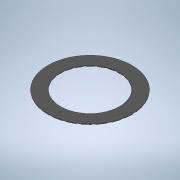
# Autodesk Inventor part: Tarcza_Okładzina_Cierna
Saved by Autodesk Inventor 2022 (Build 260153000, 153)
## iProperties
Created: 2021-06-19
Part Number: Tarcza_Okładzina_Cierna
Material: Kevlar49
Document SubType Name: Modeling
Designer: Matik
Density: 0.052 g/cm^3
Appearance: Ogólny
Author: Matik
Autodesk Inventor part; units mm, degrees
ref_plane "YZ Plane" through (0, 0, 0) normal (1, 0, 0) x (0, 1, 0)
ref_plane "XZ Plane" through (0, 0, 0) normal (0, 1, 0) x (-1, 0, 0)
ref_plane "XY Plane" through (0, 0, 0) normal (0, 0, 1) x (1, 0, 0)
sketch "Szkic1" plane through (0, 0, 0) normal (0, 1, 0) x (-1, 0, 0)
  circle A0 centre (0, 0) radius 100
  circle A1 centre (0, 0) radius 70
  line L0 (70, 0) -> (70, 5.198254)
  line L1 (70, 0) -> (70, -6.043615)
  line L2 (72.279206, 7.178669) -> (98.104364, 3.537745)
  line L3 (71.386072, -7.947058) -> (96.155566, -15.936103)
  line L4 (99.820589, 1.422211) -> (98.764925, -14.16778)
  arc A2 (72.279206, 7.178669) -> (70, 5.198254) centre (72, 5.198254) ccw
  arc A3 (70, -6.043615) -> (71.386072, -7.947058) centre (72, -6.043615) ccw
  arc A4 (96.155566, -15.936103) -> (98.764925, -14.16778) centre (96.769494, -14.032661) ccw
  arc A5 (99.820589, 1.422211) -> (98.104364, 3.537745) centre (97.825158, 1.55733) ccw
  line L5 (96.051189, 27.20922) -> (99.066483, 11.877219)
  arc A6 (96.051189, 27.20922) -> (93.845903, 28.808478) centre (94.08878, 26.82328) ccw
  line L6 (67.958375, 25.641297) -> (93.845903, 28.808478)
  arc A7 (67.958375, 25.641297) -> (66.269401, 23.138461) centre (68.201252, 23.656099) ccw
  line L7 (67.614808, 18.117333) -> (69.179011, 12.279649)
  line L8 (67.614808, 18.117333) -> (66.269401, 23.138461)
  line L9 (71.0105, 10.799807) -> (97.003712, 9.493798)
  arc A8 (69.179011, 12.279649) -> (71.0105, 10.799807) centre (71.110862, 12.797287) ccw
  arc A9 (97.003712, 9.493798) -> (99.066483, 11.877219) centre (97.104074, 11.491278) ccw
  line L10 (85.73606, 51.141966) -> (92.616824, 37.112805)
  arc A10 (85.73606, 51.141966) -> (83.191999, 52.11596) centre (83.940407, 50.261267) ccw
  line L11 (59.006294, 42.356513) -> (83.191999, 52.11596)
  arc A11 (59.006294, 42.356513) -> (58.022651, 39.50182) centre (59.754702, 40.50182) ccw
  line L12 (60.621778, 35) -> (63.643586, 29.766076)
  line L13 (60.621778, 35) -> (58.022651, 39.50182)
  line L14 (65.795681, 28.810682) -> (91.241215, 34.276713)
  arc A12 (63.643586, 29.766076) -> (65.795681, 28.810682) centre (65.375637, 30.766076) ccw
  arc A13 (91.241215, 34.276713) -> (92.616824, 37.112805) centre (90.821171, 36.232106) ccw
  line L15 (69.57816, 71.589471) -> (79.855481, 59.819215)
  arc A14 (69.57816, 71.589471) -> (66.868698, 71.871825) centre (68.071634, 70.274032) ccw
  line L16 (46.033031, 56.185202) -> (66.868698, 71.871825)
  arc A15 (46.033031, 56.185202) -> (45.821754, 53.173195) centre (47.235967, 54.587409) ccw
  line L17 (49.497475, 49.497475) -> (53.770956, 45.223993)
  line L18 (49.497475, 49.497475) -> (45.821754, 53.173195)
  line L19 (56.096994, 44.858157) -> (79.26078, 56.723726)
  arc A16 (53.770956, 45.223993) -> (56.096994, 44.858157) centre (55.18517, 46.638207) ccw
  arc A17 (79.26078, 56.723726) -> (79.855481, 59.819215) centre (78.348955, 58.503776) ccw
  line L20 (48.678623, 87.158271) -> (61.65212, 78.449044)
  arc A18 (48.678623, 87.158271) -> (45.988405, 86.729745) centre (47.563892, 85.497737) ccw
  line L21 (29.922693, 66.184963) -> (45.988405, 86.729745)
  arc A19 (29.922693, 66.184963) -> (30.49818, 63.220905) centre (31.49818, 64.952956) ccw
  line L22 (35, 60.621778) -> (40.233924, 57.599971)
  line L23 (35, 60.621778) -> (30.49818, 63.220905)
  line L24 (42.57539, 57.848623) -> (61.878853, 75.305111)
  arc A20 (40.233924, 57.599971) -> (42.57539, 57.848623) centre (41.233924, 59.332021) ccw
  arc A21 (61.878853, 75.305111) -> (61.65212, 78.449044) centre (60.537388, 76.78851) ccw
  line L25 (24.461719, 96.78738) -> (39.247268, 91.7327)
  arc A22 (24.461719, 96.78738) -> (21.974078, 95.677175) centre (23.814749, 94.894914) ccw
  line L26 (11.773173, 71.674328) -> (21.974078, 95.677175)
  arc A23 (11.773173, 71.674328) -> (13.096205, 68.960215) centre (13.613843, 70.892067) ccw
  line L27 (18.117333, 67.614808) -> (23.955017, 66.050605)
  line L28 (18.117333, 67.614808) -> (13.096205, 68.960215)
  line L29 (26.152343, 66.896801) -> (40.279986, 88.754578)
  arc A24 (23.955017, 66.050605) -> (26.152343, 66.896801) centre (24.472655, 67.982457) ccw
  arc A25 (40.279986, 88.754578) -> (39.247268, 91.7327) centre (38.600298, 89.840234) ccw
  line L30 (-1.422211, 99.820589) -> (14.16778, 98.764925)
  arc A26 (-1.422211, 99.820589) -> (-3.537745, 98.104364) centre (-1.55733, 97.825158) ccw
  line L31 (-7.178669, 72.279206) -> (-3.537745, 98.104364)
  arc A27 (-7.178669, 72.279206) -> (-5.198254, 70) centre (-5.198254, 72) ccw
  line L32 (0, 70) -> (6.043615, 70)
  line L33 (0, 70) -> (-5.198254, 70)
  line L34 (7.947058, 71.386072) -> (15.936103, 96.155566)
  arc A28 (6.043615, 70) -> (7.947058, 71.386072) centre (6.043615, 72) ccw
  arc A29 (15.936103, 96.155566) -> (14.16778, 98.764925) centre (14.032661, 96.769494) ccw
  line L35 (-27.20922, 96.051189) -> (-11.877219, 99.066483)
  arc A30 (-27.20922, 96.051189) -> (-28.808478, 93.845903) centre (-26.82328, 94.08878) ccw
  line L36 (-25.641297, 67.958375) -> (-28.808478, 93.845903)
  arc A31 (-25.641297, 67.958375) -> (-23.138461, 66.269401) centre (-23.656099, 68.201252) ccw
  line L37 (-18.117333, 67.614808) -> (-12.279649, 69.179011)
  line L38 (-18.117333, 67.614808) -> (-23.138461, 66.269401)
  line L39 (-10.799807, 71.0105) -> (-9.493798, 97.003712)
  arc A32 (-12.279649, 69.179011) -> (-10.799807, 71.0105) centre (-12.797287, 71.110862) ccw
  arc A33 (-9.493798, 97.003712) -> (-11.877219, 99.066483) centre (-11.491278, 97.104074) ccw
  line L40 (-51.141966, 85.73606) -> (-37.112805, 92.616824)
  arc A34 (-51.141966, 85.73606) -> (-52.11596, 83.191999) centre (-50.261267, 83.940407) ccw
  line L41 (-42.356513, 59.006294) -> (-52.11596, 83.191999)
  arc A35 (-42.356513, 59.006294) -> (-39.50182, 58.022651) centre (-40.50182, 59.754702) ccw
  line L42 (-35, 60.621778) -> (-29.766076, 63.643586)
  line L43 (-35, 60.621778) -> (-39.50182, 58.022651)
  line L44 (-28.810682, 65.795681) -> (-34.276713, 91.241215)
  arc A36 (-29.766076, 63.643586) -> (-28.810682, 65.795681) centre (-30.766076, 65.375637) ccw
  arc A37 (-34.276713, 91.241215) -> (-37.112805, 92.616824) centre (-36.232106, 90.821171) ccw
  line L45 (-71.589471, 69.57816) -> (-59.819215, 79.855481)
  arc A38 (-71.589471, 69.57816) -> (-71.871825, 66.868698) centre (-70.274032, 68.071634) ccw
  line L46 (-56.185202, 46.033031) -> (-71.871825, 66.868698)
  arc A39 (-56.185202, 46.033031) -> (-53.173195, 45.821754) centre (-54.587409, 47.235967) ccw
  line L47 (-49.497475, 49.497475) -> (-45.223993, 53.770956)
  line L48 (-49.497475, 49.497475) -> (-53.173195, 45.821754)
  line L49 (-44.858157, 56.096994) -> (-56.723726, 79.26078)
  arc A40 (-45.223993, 53.770956) -> (-44.858157, 56.096994) centre (-46.638207, 55.18517) ccw
  arc A41 (-56.723726, 79.26078) -> (-59.819215, 79.855481) centre (-58.503776, 78.348955) ccw
  line L50 (-87.158271, 48.678623) -> (-78.449044, 61.65212)
  arc A42 (-87.158271, 48.678623) -> (-86.729745, 45.988405) centre (-85.497737, 47.563892) ccw
  line L51 (-66.184963, 29.922693) -> (-86.729745, 45.988405)
  arc A43 (-66.184963, 29.922693) -> (-63.220905, 30.49818) centre (-64.952956, 31.49818) ccw
  line L52 (-60.621778, 35) -> (-57.599971, 40.233924)
  line L53 (-60.621778, 35) -> (-63.220905, 30.49818)
  line L54 (-57.848623, 42.57539) -> (-75.305111, 61.878853)
  arc A44 (-57.599971, 40.233924) -> (-57.848623, 42.57539) centre (-59.332021, 41.233924) ccw
  arc A45 (-75.305111, 61.878853) -> (-78.449044, 61.65212) centre (-76.78851, 60.537388) ccw
  line L55 (-96.78738, 24.461719) -> (-91.7327, 39.247268)
  arc A46 (-96.78738, 24.461719) -> (-95.677175, 21.974078) centre (-94.894914, 23.814749) ccw
  line L56 (-71.674328, 11.773173) -> (-95.677175, 21.974078)
  arc A47 (-71.674328, 11.773173) -> (-68.960215, 13.096205) centre (-70.892067, 13.613843) ccw
  line L57 (-67.614808, 18.117333) -> (-66.050605, 23.955017)
  line L58 (-67.614808, 18.117333) -> (-68.960215, 13.096205)
  line L59 (-66.896801, 26.152343) -> (-88.754578, 40.279986)
  arc A48 (-66.050605, 23.955017) -> (-66.896801, 26.152343) centre (-67.982457, 24.472655) ccw
  arc A49 (-88.754578, 40.279986) -> (-91.7327, 39.247268) centre (-89.840234, 38.600298) ccw
  line L60 (-99.820589, -1.422211) -> (-98.764925, 14.16778)
  arc A50 (-99.820589, -1.422211) -> (-98.104364, -3.537745) centre (-97.825158, -1.55733) ccw
  line L61 (-72.279206, -7.178669) -> (-98.104364, -3.537745)
  arc A51 (-72.279206, -7.178669) -> (-70, -5.198254) centre (-72, -5.198254) ccw
  line L62 (-70, 0) -> (-70, 6.043615)
  line L63 (-70, 0) -> (-70, -5.198254)
  line L64 (-71.386072, 7.947058) -> (-96.155566, 15.936103)
  arc A52 (-70, 6.043615) -> (-71.386072, 7.947058) centre (-72, 6.043615) ccw
  arc A53 (-96.155566, 15.936103) -> (-98.764925, 14.16778) centre (-96.769494, 14.032661) ccw
  line L65 (-96.051189, -27.20922) -> (-99.066483, -11.877219)
  arc A54 (-96.051189, -27.20922) -> (-93.845903, -28.808478) centre (-94.08878, -26.82328) ccw
  line L66 (-67.958375, -25.641297) -> (-93.845903, -28.808478)
  arc A55 (-67.958375, -25.641297) -> (-66.269401, -23.138461) centre (-68.201252, -23.656099) ccw
  line L67 (-67.614808, -18.117333) -> (-69.179011, -12.279649)
  line L68 (-67.614808, -18.117333) -> (-66.269401, -23.138461)
  line L69 (-71.0105, -10.799807) -> (-97.003712, -9.493798)
  arc A56 (-69.179011, -12.279649) -> (-71.0105, -10.799807) centre (-71.110862, -12.797287) ccw
  arc A57 (-97.003712, -9.493798) -> (-99.066483, -11.877219) centre (-97.104074, -11.491278) ccw
  line L70 (-85.73606, -51.141966) -> (-92.616824, -37.112805)
  arc A58 (-85.73606, -51.141966) -> (-83.191999, -52.11596) centre (-83.940407, -50.261267) ccw
  line L71 (-59.006294, -42.356513) -> (-83.191999, -52.11596)
  arc A59 (-59.006294, -42.356513) -> (-58.022651, -39.50182) centre (-59.754702, -40.50182) ccw
  line L72 (-60.621778, -35) -> (-63.643586, -29.766076)
  line L73 (-60.621778, -35) -> (-58.022651, -39.50182)
  line L74 (-65.795681, -28.810682) -> (-91.241215, -34.276713)
  arc A60 (-63.643586, -29.766076) -> (-65.795681, -28.810682) centre (-65.375637, -30.766076) ccw
  arc A61 (-91.241215, -34.276713) -> (-92.616824, -37.112805) centre (-90.821171, -36.232106) ccw
  line L75 (-69.57816, -71.589471) -> (-79.855481, -59.819215)
  arc A62 (-69.57816, -71.589471) -> (-66.868698, -71.871825) centre (-68.071634, -70.274032) ccw
  line L76 (-46.033031, -56.185202) -> (-66.868698, -71.871825)
  arc A63 (-46.033031, -56.185202) -> (-45.821754, -53.173195) centre (-47.235967, -54.587409) ccw
  line L77 (-49.497475, -49.497475) -> (-53.770956, -45.223993)
  line L78 (-49.497475, -49.497475) -> (-45.821754, -53.173195)
  line L79 (-56.096994, -44.858157) -> (-79.26078, -56.723726)
  arc A64 (-53.770956, -45.223993) -> (-56.096994, -44.858157) centre (-55.18517, -46.638207) ccw
  arc A65 (-79.26078, -56.723726) -> (-79.855481, -59.819215) centre (-78.348955, -58.503776) ccw
  line L80 (-48.678623, -87.158271) -> (-61.65212, -78.449044)
  arc A66 (-48.678623, -87.158271) -> (-45.988405, -86.729745) centre (-47.563892, -85.497737) ccw
  line L81 (-29.922693, -66.184963) -> (-45.988405, -86.729745)
  arc A67 (-29.922693, -66.184963) -> (-30.49818, -63.220905) centre (-31.49818, -64.952956) ccw
  line L82 (-35, -60.621778) -> (-40.233924, -57.599971)
  line L83 (-35, -60.621778) -> (-30.49818, -63.220905)
  line L84 (-42.57539, -57.848623) -> (-61.878853, -75.305111)
  arc A68 (-40.233924, -57.599971) -> (-42.57539, -57.848623) centre (-41.233924, -59.332021) ccw
  arc A69 (-61.878853, -75.305111) -> (-61.65212, -78.449044) centre (-60.537388, -76.78851) ccw
  line L85 (-24.461719, -96.78738) -> (-39.247268, -91.7327)
  arc A70 (-24.461719, -96.78738) -> (-21.974078, -95.677175) centre (-23.814749, -94.894914) ccw
  line L86 (-11.773173, -71.674328) -> (-21.974078, -95.677175)
  arc A71 (-11.773173, -71.674328) -> (-13.096205, -68.960215) centre (-13.613843, -70.892067) ccw
  line L87 (-18.117333, -67.614808) -> (-23.955017, -66.050605)
  line L88 (-18.117333, -67.614808) -> (-13.096205, -68.960215)
  line L89 (-26.152343, -66.896801) -> (-40.279986, -88.754578)
  arc A72 (-23.955017, -66.050605) -> (-26.152343, -66.896801) centre (-24.472655, -67.982457) ccw
  arc A73 (-40.279986, -88.754578) -> (-39.247268, -91.7327) centre (-38.600298, -89.840234) ccw
  line L90 (1.422211, -99.820589) -> (-14.16778, -98.764925)
  arc A74 (1.422211, -99.820589) -> (3.537745, -98.104364) centre (1.55733, -97.825158) ccw
  line L91 (7.178669, -72.279206) -> (3.537745, -98.104364)
  arc A75 (7.178669, -72.279206) -> (5.198254, -70) centre (5.198254, -72) ccw
  line L92 (0, -70) -> (-6.043615, -70)
  line L93 (0, -70) -> (5.198254, -70)
  line L94 (-7.947058, -71.386072) -> (-15.936103, -96.155566)
  arc A76 (-6.043615, -70) -> (-7.947058, -71.386072) centre (-6.043615, -72) ccw
  arc A77 (-15.936103, -96.155566) -> (-14.16778, -98.764925) centre (-14.032661, -96.769494) ccw
  line L95 (27.20922, -96.051189) -> (11.877219, -99.066483)
  arc A78 (27.20922, -96.051189) -> (28.808478, -93.845903) centre (26.82328, -94.08878) ccw
  line L96 (25.641297, -67.958375) -> (28.808478, -93.845903)
  arc A79 (25.641297, -67.958375) -> (23.138461, -66.269401) centre (23.656099, -68.201252) ccw
  line L97 (18.117333, -67.614808) -> (12.279649, -69.179011)
  line L98 (18.117333, -67.614808) -> (23.138461, -66.269401)
  line L99 (10.799807, -71.0105) -> (9.493798, -97.003712)
  arc A80 (12.279649, -69.179011) -> (10.799807, -71.0105) centre (12.797287, -71.110862) ccw
  arc A81 (9.493798, -97.003712) -> (11.877219, -99.066483) centre (11.491278, -97.104074) ccw
  line L100 (51.141966, -85.73606) -> (37.112805, -92.616824)
  arc A82 (51.141966, -85.73606) -> (52.11596, -83.191999) centre (50.261267, -83.940407) ccw
  line L101 (42.356513, -59.006294) -> (52.11596, -83.191999)
  arc A83 (42.356513, -59.006294) -> (39.50182, -58.022651) centre (40.50182, -59.754702) ccw
  line L102 (35, -60.621778) -> (29.766076, -63.643586)
  line L103 (35, -60.621778) -> (39.50182, -58.022651)
  line L104 (28.810682, -65.795681) -> (34.276713, -91.241215)
  arc A84 (29.766076, -63.643586) -> (28.810682, -65.795681) centre (30.766076, -65.375637) ccw
  arc A85 (34.276713, -91.241215) -> (37.112805, -92.616824) centre (36.232106, -90.821171) ccw
  line L105 (71.589471, -69.57816) -> (59.819215, -79.855481)
  arc A86 (71.589471, -69.57816) -> (71.871825, -66.868698) centre (70.274032, -68.071634) ccw
  line L106 (56.185202, -46.033031) -> (71.871825, -66.868698)
  arc A87 (56.185202, -46.033031) -> (53.173195, -45.821754) centre (54.587409, -47.235967) ccw
  line L107 (49.497475, -49.497475) -> (45.223993, -53.770956)
  line L108 (49.497475, -49.497475) -> (53.173195, -45.821754)
  line L109 (44.858157, -56.096994) -> (56.723726, -79.26078)
  arc A88 (45.223993, -53.770956) -> (44.858157, -56.096994) centre (46.638207, -55.18517) ccw
  arc A89 (56.723726, -79.26078) -> (59.819215, -79.855481) centre (58.503776, -78.348955) ccw
  line L110 (87.158271, -48.678623) -> (78.449044, -61.65212)
  arc A90 (87.158271, -48.678623) -> (86.729745, -45.988405) centre (85.497737, -47.563892) ccw
  line L111 (66.184963, -29.922693) -> (86.729745, -45.988405)
  arc A91 (66.184963, -29.922693) -> (63.220905, -30.49818) centre (64.952956, -31.49818) ccw
  line L112 (60.621778, -35) -> (57.599971, -40.233924)
  line L113 (60.621778, -35) -> (63.220905, -30.49818)
  line L114 (57.848623, -42.57539) -> (75.305111, -61.878853)
  arc A92 (57.599971, -40.233924) -> (57.848623, -42.57539) centre (59.332021, -41.233924) ccw
  arc A93 (75.305111, -61.878853) -> (78.449044, -61.65212) centre (76.78851, -60.537388) ccw
  line L115 (96.78738, -24.461719) -> (91.7327, -39.247268)
  arc A94 (96.78738, -24.461719) -> (95.677175, -21.974078) centre (94.894914, -23.814749) ccw
  line L116 (71.674328, -11.773173) -> (95.677175, -21.974078)
  arc A95 (71.674328, -11.773173) -> (68.960215, -13.096205) centre (70.892067, -13.613843) ccw
  line L117 (67.614808, -18.117333) -> (66.050605, -23.955017)
  line L118 (67.614808, -18.117333) -> (68.960215, -13.096205)
  line L119 (66.896801, -26.152343) -> (88.754578, -40.279986)
  arc A96 (66.050605, -23.955017) -> (66.896801, -26.152343) centre (67.982457, -24.472655) ccw
  arc A97 (88.754578, -40.279986) -> (91.7327, -39.247268) centre (89.840234, -38.600298) ccw
  point P0 (70, 7.5)
  point P1 (70, -7.5)
  point P2 (99.946257, 3.278069)
  point P3 (98.591972, -16.721931)
  point P4 (98.591972, -16.721931)
  point P5 (99.560487, 9.365335)
  point P6 (95.692244, 29.034366)
  point P7 (65.673665, 25.361777)
  point P8 (69.555951, 10.872889)
  point P9 (99.560487, 9.365335)
  point P10 (93.744118, 34.814369)
  point P11 (84.916963, 52.812019)
  point P12 (56.871778, 41.495191)
  point P13 (64.371778, 28.504809)
  point P14 (93.744118, 34.814369)
  point P15 (81.539243, 57.890861)
  point P16 (68.354731, 72.990621)
  point P17 (44.194174, 54.800776)
  point P18 (54.800776, 44.194174)
  point P19 (81.539243, 57.890861)
  point P20 (63.777603, 77.022187)
  point P21 (47.134238, 88.195032)
  point P22 (28.504809, 64.371778)
  point P23 (41.495191, 56.871778)
  point P24 (63.777603, 77.022187)
  point P25 (41.669625, 90.904578)
  point P26 (22.701623, 97.389097)
  point P27 (10.872889, 69.555951)
  point P28 (25.361777, 65.673665)
  point P29 (41.669625, 90.904578)
  point P30 (16.721931, 98.591972)
  point P31 (-3.278069, 99.946257)
  point P32 (-7.5, 70)
  point P33 (7.5, 70)
  point P34 (16.721931, 98.591972)
  point P35 (-9.365335, 99.560487)
  point P36 (-29.034366, 95.692244)
  point P37 (-25.361777, 65.673665)
  point P38 (-10.872889, 69.555951)
  point P39 (-9.365335, 99.560487)
  point P40 (-34.814369, 93.744118)
  point P41 (-52.812019, 84.916963)
  point P42 (-41.495191, 56.871778)
  point P43 (-28.504809, 64.371778)
  point P44 (-34.814369, 93.744118)
  point P45 (-57.890861, 81.539243)
  point P46 (-72.990621, 68.354731)
  point P47 (-54.800776, 44.194174)
  point P48 (-44.194174, 54.800776)
  point P49 (-57.890861, 81.539243)
  point P50 (-77.022187, 63.777603)
  point P51 (-88.195032, 47.134238)
  point P52 (-64.371778, 28.504809)
  point P53 (-56.871778, 41.495191)
  point P54 (-77.022187, 63.777603)
  point P55 (-90.904578, 41.669625)
  point P56 (-97.389097, 22.701623)
  point P57 (-69.555951, 10.872889)
  point P58 (-65.673665, 25.361777)
  point P59 (-90.904578, 41.669625)
  point P60 (-98.591972, 16.721931)
  point P61 (-99.946257, -3.278069)
  point P62 (-70, -7.5)
  point P63 (-70, 7.5)
  point P64 (-98.591972, 16.721931)
  point P65 (-99.560487, -9.365335)
  point P66 (-95.692244, -29.034366)
  point P67 (-65.673665, -25.361777)
  point P68 (-69.555951, -10.872889)
  point P69 (-99.560487, -9.365335)
  point P70 (-93.744118, -34.814369)
  point P71 (-84.916963, -52.812019)
  point P72 (-56.871778, -41.495191)
  point P73 (-64.371778, -28.504809)
  point P74 (-93.744118, -34.814369)
  point P75 (-81.539243, -57.890861)
  point P76 (-68.354731, -72.990621)
  point P77 (-44.194174, -54.800776)
  point P78 (-54.800776, -44.194174)
  point P79 (-81.539243, -57.890861)
  point P80 (-63.777603, -77.022187)
  point P81 (-47.134238, -88.195032)
  point P82 (-28.504809, -64.371778)
  point P83 (-41.495191, -56.871778)
  point P84 (-63.777603, -77.022187)
  point P85 (-41.669625, -90.904578)
  point P86 (-22.701623, -97.389097)
  point P87 (-10.872889, -69.555951)
  point P88 (-25.361777, -65.673665)
  point P89 (-41.669625, -90.904578)
  point P90 (-16.721931, -98.591972)
  point P91 (3.278069, -99.946257)
  point P92 (7.5, -70)
  point P93 (-7.5, -70)
  point P94 (-16.721931, -98.591972)
  point P95 (9.365335, -99.560487)
  point P96 (29.034366, -95.692244)
  point P97 (25.361777, -65.673665)
  point P98 (10.872889, -69.555951)
  point P99 (9.365335, -99.560487)
  point P100 (34.814369, -93.744118)
  point P101 (52.812019, -84.916963)
  point P102 (41.495191, -56.871778)
  point P103 (28.504809, -64.371778)
  point P104 (34.814369, -93.744118)
  point P105 (57.890861, -81.539243)
  point P106 (72.990621, -68.354731)
  point P107 (54.800776, -44.194174)
  point P108 (44.194174, -54.800776)
  point P109 (57.890861, -81.539243)
  point P110 (77.022187, -63.777603)
  point P111 (88.195032, -47.134238)
  point P112 (64.371778, -28.504809)
  point P113 (56.871778, -41.495191)
  point P114 (77.022187, -63.777603)
  point P115 (90.904578, -41.669625)
  point P116 (97.389097, -22.701623)
  point P117 (69.555951, -10.872889)
  point P118 (65.673665, -25.361777)
  point P119 (90.904578, -41.669625)
  dimension "d1" = 140
  dimension "d0" = 200
  dimension "d3" = 7.5
  dimension "d4" = 7.5
  dimension "d7" = 20
  dimension "d8" = 2
  dimension "d11" = 360
  constraints: 240 end point, 216 point on line, 195 point on circle, 97 centre point, 8 tangent, 3 equal radius, 2 coincident, 2 vertical, 1 horizontal alignment, 651 other
  measures "d0" diameter of A0
  measures "d3" distance of L0.start point (70, 7.5)
  measures "d4" distance of L0.start point (70, -7.5)
  measures "d7" vertical distance of point (98.592, -16.722) A0.start
  measures "d8" radius of A2
sketch "Szkic1 outline for Wyciągnięcie proste1" plane through (0, 0, 0) normal (0, 1, 0) x (-1, 0, 0)
  arc A0 (69.179011, 12.279649) -> (71.0105, 10.799807) centre (71.110862, 12.797287) ccw
  line L0 (71.0105, 10.799807) -> (97.003712, 9.493798)
  arc A1 (97.003712, 9.493798) -> (99.066483, 11.877219) centre (97.104074, 11.491278) ccw
  line L1 (99.066483, 11.877219) -> (96.051189, 27.20922)
  arc A2 (96.051189, 27.20922) -> (93.845903, 28.808478) centre (94.08878, 26.82328) ccw
  line L2 (93.845903, 28.808478) -> (67.958375, 25.641297)
  arc A3 (67.958375, 25.641297) -> (66.269401, 23.138461) centre (68.201252, 23.656099) ccw
  line L3 (66.269401, 23.138461) -> (69.179011, 12.279649)
  arc A4 (63.643586, 29.766076) -> (65.795681, 28.810682) centre (65.375637, 30.766076) ccw
  line L4 (65.795681, 28.810682) -> (91.241215, 34.276713)
  arc A5 (91.241215, 34.276713) -> (92.616824, 37.112805) centre (90.821171, 36.232106) ccw
  line L5 (92.616824, 37.112805) -> (85.73606, 51.141966)
  arc A6 (85.73606, 51.141966) -> (83.191999, 52.11596) centre (83.940407, 50.261267) ccw
  line L6 (83.191999, 52.11596) -> (59.006294, 42.356513)
  arc A7 (59.006294, 42.356513) -> (58.022651, 39.50182) centre (59.754702, 40.50182) ccw
  line L7 (58.022651, 39.50182) -> (63.643586, 29.766076)
  arc A8 (53.770956, 45.223993) -> (56.096994, 44.858157) centre (55.18517, 46.638207) ccw
  line L8 (56.096994, 44.858157) -> (79.26078, 56.723726)
  arc A9 (79.26078, 56.723726) -> (79.855481, 59.819215) centre (78.348955, 58.503776) ccw
  line L9 (79.855481, 59.819215) -> (69.57816, 71.589471)
  arc A10 (69.57816, 71.589471) -> (66.868698, 71.871825) centre (68.071634, 70.274032) ccw
  line L10 (66.868698, 71.871825) -> (46.033031, 56.185202)
  arc A11 (46.033031, 56.185202) -> (45.821754, 53.173195) centre (47.235967, 54.587409) ccw
  line L11 (45.821754, 53.173195) -> (53.770956, 45.223993)
  arc A12 (40.233924, 57.599971) -> (42.57539, 57.848623) centre (41.233924, 59.332021) ccw
  line L12 (42.57539, 57.848623) -> (61.878853, 75.305111)
  arc A13 (61.878853, 75.305111) -> (61.65212, 78.449044) centre (60.537388, 76.78851) ccw
  line L13 (61.65212, 78.449044) -> (48.678623, 87.158271)
  arc A14 (48.678623, 87.158271) -> (45.988405, 86.729745) centre (47.563892, 85.497737) ccw
  line L14 (45.988405, 86.729745) -> (29.922693, 66.184963)
  arc A15 (29.922693, 66.184963) -> (30.49818, 63.220905) centre (31.49818, 64.952956) ccw
  line L15 (30.49818, 63.220905) -> (40.233924, 57.599971)
  arc A16 (23.955017, 66.050605) -> (26.152343, 66.896801) centre (24.472655, 67.982457) ccw
  line L16 (26.152343, 66.896801) -> (40.279986, 88.754578)
  arc A17 (40.279986, 88.754578) -> (39.247268, 91.7327) centre (38.600298, 89.840234) ccw
  line L17 (39.247268, 91.7327) -> (24.461719, 96.78738)
  arc A18 (24.461719, 96.78738) -> (21.974078, 95.677175) centre (23.814749, 94.894914) ccw
  line L18 (21.974078, 95.677175) -> (11.773173, 71.674328)
  arc A19 (11.773173, 71.674328) -> (13.096205, 68.960215) centre (13.613843, 70.892067) ccw
  line L19 (13.096205, 68.960215) -> (23.955017, 66.050605)
  arc A20 (6.043615, 70) -> (7.947058, 71.386072) centre (6.043615, 72) ccw
  line L20 (7.947058, 71.386072) -> (15.936103, 96.155566)
  arc A21 (15.936103, 96.155566) -> (14.16778, 98.764925) centre (14.032661, 96.769494) ccw
  line L21 (14.16778, 98.764925) -> (-1.422211, 99.820589)
  arc A22 (-1.422211, 99.820589) -> (-3.537745, 98.104364) centre (-1.55733, 97.825158) ccw
  line L22 (-3.537745, 98.104364) -> (-7.178669, 72.279206)
  arc A23 (-7.178669, 72.279206) -> (-5.198254, 70) centre (-5.198254, 72) ccw
  line L23 (-5.198254, 70) -> (6.043615, 70)
  arc A24 (-12.279649, 69.179011) -> (-10.799807, 71.0105) centre (-12.797287, 71.110862) ccw
  line L24 (-10.799807, 71.0105) -> (-9.493798, 97.003712)
  arc A25 (-9.493798, 97.003712) -> (-11.877219, 99.066483) centre (-11.491278, 97.104074) ccw
  line L25 (-11.877219, 99.066483) -> (-27.20922, 96.051189)
  arc A26 (-27.20922, 96.051189) -> (-28.808478, 93.845903) centre (-26.82328, 94.08878) ccw
  line L26 (-28.808478, 93.845903) -> (-25.641297, 67.958375)
  arc A27 (-25.641297, 67.958375) -> (-23.138461, 66.269401) centre (-23.656099, 68.201252) ccw
  line L27 (-23.138461, 66.269401) -> (-12.279649, 69.179011)
  arc A28 (-29.766076, 63.643586) -> (-28.810682, 65.795681) centre (-30.766076, 65.375637) ccw
  line L28 (-28.810682, 65.795681) -> (-34.276713, 91.241215)
  arc A29 (-34.276713, 91.241215) -> (-37.112805, 92.616824) centre (-36.232106, 90.821171) ccw
  line L29 (-37.112805, 92.616824) -> (-51.141966, 85.73606)
  arc A30 (-51.141966, 85.73606) -> (-52.11596, 83.191999) centre (-50.261267, 83.940407) ccw
  line L30 (-52.11596, 83.191999) -> (-42.356513, 59.006294)
  arc A31 (-42.356513, 59.006294) -> (-39.50182, 58.022651) centre (-40.50182, 59.754702) ccw
  line L31 (-39.50182, 58.022651) -> (-29.766076, 63.643586)
  arc A32 (-57.599971, 40.233924) -> (-57.848623, 42.57539) centre (-59.332021, 41.233924) ccw
  line L32 (-57.848623, 42.57539) -> (-75.305111, 61.878853)
  arc A33 (-75.305111, 61.878853) -> (-78.449044, 61.65212) centre (-76.78851, 60.537388) ccw
  line L33 (-78.449044, 61.65212) -> (-87.158271, 48.678623)
  arc A34 (-87.158271, 48.678623) -> (-86.729745, 45.988405) centre (-85.497737, 47.563892) ccw
  line L34 (-86.729745, 45.988405) -> (-66.184963, 29.922693)
  arc A35 (-66.184963, 29.922693) -> (-63.220905, 30.49818) centre (-64.952956, 31.49818) ccw
  line L35 (-63.220905, 30.49818) -> (-57.599971, 40.233924)
  arc A36 (-45.223993, 53.770956) -> (-44.858157, 56.096994) centre (-46.638207, 55.18517) ccw
  line L36 (-44.858157, 56.096994) -> (-56.723726, 79.26078)
  arc A37 (-56.723726, 79.26078) -> (-59.819215, 79.855481) centre (-58.503776, 78.348955) ccw
  line L37 (-59.819215, 79.855481) -> (-71.589471, 69.57816)
  arc A38 (-71.589471, 69.57816) -> (-71.871825, 66.868698) centre (-70.274032, 68.071634) ccw
  line L38 (-71.871825, 66.868698) -> (-56.185202, 46.033031)
  arc A39 (-56.185202, 46.033031) -> (-53.173195, 45.821754) centre (-54.587409, 47.235967) ccw
  line L39 (-53.173195, 45.821754) -> (-45.223993, 53.770956)
  arc A40 (-66.050605, 23.955017) -> (-66.896801, 26.152343) centre (-67.982457, 24.472655) ccw
  line L40 (-66.896801, 26.152343) -> (-88.754578, 40.279986)
  arc A41 (-88.754578, 40.279986) -> (-91.7327, 39.247268) centre (-89.840234, 38.600298) ccw
  line L41 (-91.7327, 39.247268) -> (-96.78738, 24.461719)
  arc A42 (-96.78738, 24.461719) -> (-95.677175, 21.974078) centre (-94.894914, 23.814749) ccw
  line L42 (-95.677175, 21.974078) -> (-71.674328, 11.773173)
  arc A43 (-71.674328, 11.773173) -> (-68.960215, 13.096205) centre (-70.892067, 13.613843) ccw
  line L43 (-68.960215, 13.096205) -> (-66.050605, 23.955017)
  arc A44 (-70, 6.043615) -> (-71.386072, 7.947058) centre (-72, 6.043615) ccw
  line L44 (-71.386072, 7.947058) -> (-96.155566, 15.936103)
  arc A45 (-96.155566, 15.936103) -> (-98.764925, 14.16778) centre (-96.769494, 14.032661) ccw
  line L45 (-98.764925, 14.16778) -> (-99.820589, -1.422211)
  arc A46 (-99.820589, -1.422211) -> (-98.104364, -3.537745) centre (-97.825158, -1.55733) ccw
  line L46 (-98.104364, -3.537745) -> (-72.279206, -7.178669)
  arc A47 (-72.279206, -7.178669) -> (-70, -5.198254) centre (-72, -5.198254) ccw
  line L47 (-70, -5.198254) -> (-70, 6.043615)
  arc A48 (-69.179011, -12.279649) -> (-71.0105, -10.799807) centre (-71.110862, -12.797287) ccw
  line L48 (-71.0105, -10.799807) -> (-97.003712, -9.493798)
  arc A49 (-97.003712, -9.493798) -> (-99.066483, -11.877219) centre (-97.104074, -11.491278) ccw
  line L49 (-99.066483, -11.877219) -> (-96.051189, -27.20922)
  arc A50 (-96.051189, -27.20922) -> (-93.845903, -28.808478) centre (-94.08878, -26.82328) ccw
  line L50 (-93.845903, -28.808478) -> (-67.958375, -25.641297)
  arc A51 (-67.958375, -25.641297) -> (-66.269401, -23.138461) centre (-68.201252, -23.656099) ccw
  line L51 (-66.269401, -23.138461) -> (-69.179011, -12.279649)
  arc A52 (-63.643586, -29.766076) -> (-65.795681, -28.810682) centre (-65.375637, -30.766076) ccw
  line L52 (-65.795681, -28.810682) -> (-91.241215, -34.276713)
  arc A53 (-91.241215, -34.276713) -> (-92.616824, -37.112805) centre (-90.821171, -36.232106) ccw
  line L53 (-92.616824, -37.112805) -> (-85.73606, -51.141966)
  arc A54 (-85.73606, -51.141966) -> (-83.191999, -52.11596) centre (-83.940407, -50.261267) ccw
  line L54 (-83.191999, -52.11596) -> (-59.006294, -42.356513)
  arc A55 (-59.006294, -42.356513) -> (-58.022651, -39.50182) centre (-59.754702, -40.50182) ccw
  line L55 (-58.022651, -39.50182) -> (-63.643586, -29.766076)
  arc A56 (-53.770956, -45.223993) -> (-56.096994, -44.858157) centre (-55.18517, -46.638207) ccw
  line L56 (-56.096994, -44.858157) -> (-79.26078, -56.723726)
  arc A57 (-79.26078, -56.723726) -> (-79.855481, -59.819215) centre (-78.348955, -58.503776) ccw
  line L57 (-79.855481, -59.819215) -> (-69.57816, -71.589471)
  arc A58 (-69.57816, -71.589471) -> (-66.868698, -71.871825) centre (-68.071634, -70.274032) ccw
  line L58 (-66.868698, -71.871825) -> (-46.033031, -56.185202)
  arc A59 (-46.033031, -56.185202) -> (-45.821754, -53.173195) centre (-47.235967, -54.587409) ccw
  line L59 (-45.821754, -53.173195) -> (-53.770956, -45.223993)
  arc A60 (-40.233924, -57.599971) -> (-42.57539, -57.848623) centre (-41.233924, -59.332021) ccw
  line L60 (-42.57539, -57.848623) -> (-61.878853, -75.305111)
  arc A61 (-61.878853, -75.305111) -> (-61.65212, -78.449044) centre (-60.537388, -76.78851) ccw
  line L61 (-61.65212, -78.449044) -> (-48.678623, -87.158271)
  arc A62 (-48.678623, -87.158271) -> (-45.988405, -86.729745) centre (-47.563892, -85.497737) ccw
  line L62 (-45.988405, -86.729745) -> (-29.922693, -66.184963)
  arc A63 (-29.922693, -66.184963) -> (-30.49818, -63.220905) centre (-31.49818, -64.952956) ccw
  line L63 (-30.49818, -63.220905) -> (-40.233924, -57.599971)
  arc A64 (-23.955017, -66.050605) -> (-26.152343, -66.896801) centre (-24.472655, -67.982457) ccw
  line L64 (-26.152343, -66.896801) -> (-40.279986, -88.754578)
  arc A65 (-40.279986, -88.754578) -> (-39.247268, -91.7327) centre (-38.600298, -89.840234) ccw
  line L65 (-39.247268, -91.7327) -> (-24.461719, -96.78738)
  arc A66 (-24.461719, -96.78738) -> (-21.974078, -95.677175) centre (-23.814749, -94.894914) ccw
  line L66 (-21.974078, -95.677175) -> (-11.773173, -71.674328)
  arc A67 (-11.773173, -71.674328) -> (-13.096205, -68.960215) centre (-13.613843, -70.892067) ccw
  line L67 (-13.096205, -68.960215) -> (-23.955017, -66.050605)
  arc A68 (-6.043615, -70) -> (-7.947058, -71.386072) centre (-6.043615, -72) ccw
  line L68 (-7.947058, -71.386072) -> (-15.936103, -96.155566)
  arc A69 (-15.936103, -96.155566) -> (-14.16778, -98.764925) centre (-14.032661, -96.769494) ccw
  line L69 (-14.16778, -98.764925) -> (1.422211, -99.820589)
  arc A70 (1.422211, -99.820589) -> (3.537745, -98.104364) centre (1.55733, -97.825158) ccw
  line L70 (3.537745, -98.104364) -> (7.178669, -72.279206)
  arc A71 (7.178669, -72.279206) -> (5.198254, -70) centre (5.198254, -72) ccw
  line L71 (5.198254, -70) -> (-6.043615, -70)
  arc A72 (12.279649, -69.179011) -> (10.799807, -71.0105) centre (12.797287, -71.110862) ccw
  line L72 (10.799807, -71.0105) -> (9.493798, -97.003712)
  arc A73 (9.493798, -97.003712) -> (11.877219, -99.066483) centre (11.491278, -97.104074) ccw
  line L73 (11.877219, -99.066483) -> (27.20922, -96.051189)
  arc A74 (27.20922, -96.051189) -> (28.808478, -93.845903) centre (26.82328, -94.08878) ccw
  line L74 (28.808478, -93.845903) -> (25.641297, -67.958375)
  arc A75 (25.641297, -67.958375) -> (23.138461, -66.269401) centre (23.656099, -68.201252) ccw
  line L75 (23.138461, -66.269401) -> (12.279649, -69.179011)
  arc A76 (29.766076, -63.643586) -> (28.810682, -65.795681) centre (30.766076, -65.375637) ccw
  line L76 (28.810682, -65.795681) -> (34.276713, -91.241215)
  arc A77 (34.276713, -91.241215) -> (37.112805, -92.616824) centre (36.232106, -90.821171) ccw
  line L77 (37.112805, -92.616824) -> (51.141966, -85.73606)
  arc A78 (51.141966, -85.73606) -> (52.11596, -83.191999) centre (50.261267, -83.940407) ccw
  line L78 (52.11596, -83.191999) -> (42.356513, -59.006294)
  arc A79 (42.356513, -59.006294) -> (39.50182, -58.022651) centre (40.50182, -59.754702) ccw
  line L79 (39.50182, -58.022651) -> (29.766076, -63.643586)
  arc A80 (45.223993, -53.770956) -> (44.858157, -56.096994) centre (46.638207, -55.18517) ccw
  line L80 (44.858157, -56.096994) -> (56.723726, -79.26078)
  arc A81 (56.723726, -79.26078) -> (59.819215, -79.855481) centre (58.503776, -78.348955) ccw
  line L81 (59.819215, -79.855481) -> (71.589471, -69.57816)
  arc A82 (71.589471, -69.57816) -> (71.871825, -66.868698) centre (70.274032, -68.071634) ccw
  line L82 (71.871825, -66.868698) -> (56.185202, -46.033031)
  arc A83 (56.185202, -46.033031) -> (53.173195, -45.821754) centre (54.587409, -47.235967) ccw
  line L83 (53.173195, -45.821754) -> (45.223993, -53.770956)
  arc A84 (57.599971, -40.233924) -> (57.848623, -42.57539) centre (59.332021, -41.233924) ccw
  line L84 (57.848623, -42.57539) -> (75.305111, -61.878853)
  arc A85 (75.305111, -61.878853) -> (78.449044, -61.65212) centre (76.78851, -60.537388) ccw
  line L85 (78.449044, -61.65212) -> (87.158271, -48.678623)
  arc A86 (87.158271, -48.678623) -> (86.729745, -45.988405) centre (85.497737, -47.563892) ccw
  line L86 (86.729745, -45.988405) -> (66.184963, -29.922693)
  arc A87 (66.184963, -29.922693) -> (63.220905, -30.49818) centre (64.952956, -31.49818) ccw
  line L87 (63.220905, -30.49818) -> (57.599971, -40.233924)
  arc A88 (66.050605, -23.955017) -> (66.896801, -26.152343) centre (67.982457, -24.472655) ccw
  line L88 (66.896801, -26.152343) -> (88.754578, -40.279986)
  arc A89 (88.754578, -40.279986) -> (91.7327, -39.247268) centre (89.840234, -38.600298) ccw
  line L89 (91.7327, -39.247268) -> (96.78738, -24.461719)
  arc A90 (96.78738, -24.461719) -> (95.677175, -21.974078) centre (94.894914, -23.814749) ccw
  line L90 (95.677175, -21.974078) -> (71.674328, -11.773173)
  arc A91 (71.674328, -11.773173) -> (68.960215, -13.096205) centre (70.892067, -13.613843) ccw
  line L91 (68.960215, -13.096205) -> (66.050605, -23.955017)
  line L92 (70, 5.198254) -> (70, -6.043615)
  arc A92 (70, -6.043615) -> (71.386072, -7.947058) centre (72, -6.043615) ccw
  line L93 (71.386072, -7.947058) -> (96.155566, -15.936103)
  arc A93 (96.155566, -15.936103) -> (98.764925, -14.16778) centre (96.769494, -14.032661) ccw
  line L94 (98.764925, -14.16778) -> (99.820589, 1.422211)
  arc A94 (99.820589, 1.422211) -> (98.104364, 3.537745) centre (97.825158, 1.55733) ccw
  line L95 (98.104364, 3.537745) -> (72.279206, 7.178669)
  arc A95 (72.279206, 7.178669) -> (70, 5.198254) centre (72, 5.198254) ccw
extrude "Wyciągnięcie proste1" add sketch "Szkic1 outline for Wyciągnięcie proste1" against normal blind 2
sketch "Szkic1 outline for Wyciągnięcie proste2" plane through (0, 0, 0) normal (0, 1, 0) x (-1, 0, 0)
  circle A0 centre (0, 0) radius 100
  circle A1 centre (0, 0) radius 70
extrude "Wyciągnięcie proste2" add sketch "Szkic1 outline for Wyciągnięcie proste2" against normal blind 1
